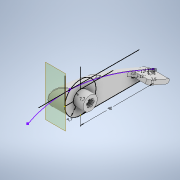
# Autodesk Inventor part: rachag2
Saved by Autodesk Inventor 2020 (Build 240168000, 168)
## iProperties
Created: 2023-10-21
Part Number: rachag2
Material: Типовые
Document SubType Name: Modeling
Designer: 522
Density: 1 g/cm^3
Appearance: По умолчанию
Author: 522
Autodesk Inventor part; units mm, degrees
ref_plane "YZ Plane" through (0, 0, 0) normal (1, 0, 0) x (0, 1, 0)
ref_plane "XZ Plane" through (0, 0, 0) normal (0, 1, 0) x (-1, 0, 0)
ref_plane "XY Plane" through (0, 0, 0) normal (0, 0, 1) x (1, 0, 0)
sketch "Эскиз1" plane through (0, 0, 0) normal (1, 0, 0) x (0, 1, 0)
  circle A0 centre (0, 0) radius 3.85
  circle A1 centre (0, 0) radius 8.55
  line L0 (-8.55, 0) -> (-8.55, -40)
  line L1 (6.55, 5.6577) -> (6.55, -32.1821)
  line L2 (3.85, 0) -> (3.85, -17.9751)
  line L3 (0, 0) -> (14.53, 0)
  line L4 (0, 0) -> (0, 8.55)
  line L5 (14.53, 8.55) -> (0, 8.55)
  arc A2 (-5.4255, -37.1668) -> (-6.7329, -39.9987) centre (-6.8, -38.25) ccw
  line L6 (6.55, 1.7425) -> (6.55, 23.1247)
  spline S0 degree 2 poles (-6.7329, -39.9987) (14.5192, 5.2155) (1.7917, 28.8286) knots 0 0 0 1 1 1
  line L7 (-6.8, -38.25) -> (-7.9249, -39.5906)
  line L8 (-6.8, -38.25) -> (-5.05, -38.25) construction
  line L9 (-1.9372, -28.9987) -> (-3.8265, -28.3121)
  line L10 (-1.9372, -28.9987) -> (-4.0049, -28.2473)
  line L11 (-6.7329, -39.9987) -> (-8.496, -38.6813)
  line L12 (-8.496, -38.6813) -> (-4.0049, -28.2473)
  point P0 (5.9063, 6.1821)
  point P1 (6.505, 5.5486)
  point P2 (-8.55, -38.25)
  point P3 (3.85, -11.5167)
  point P4 (3.85, -7.6341)
  point P5 (4.8879, -7.0151)
  dimension "d0" = 7.7
  dimension "d1" = 4.7
  dimension "d4" = 2.7
  dimension "d100" = 40
  dimension "d101" = 3.5
  dimension "d102" = 1.75
  dimension "d103" = 1.75
  dimension "d113" = 1.75
  dimension "d114" = 130
  dimension "d115" = 12
  dimension "d116" = 12
  dimension "d117" = 2.2
  constraints: 26 end point, 7 point on circle, 6 vertical, 2 centre point, 2 coincident, 2 horizontal, 2 point on line, 2 tangent, 1 equal length, 1 horizontal alignment, 1 perpendicular, 8 other
  measures "d4" distance between parallel lines of L2 L1
  measures "d100" distance of L0.start L0.end
  measures "d101" diameter of A2
  measures "d102" horizontal distance of L0.end L7.start
  measures "d103" horizontal distance of L0.end L7.start
  measures "d113" distance of L7.start L7.end
  measures "d114" angle of L7 L8
  measures "d115" distance of L7.end L9.end
  measures "d116" distance of L11.start L9.start
  measures "d117" distance of L9.start L10.end
extrude "Выдавливание1" add sketch "Эскиз1" against normal blind 10 contours L3 L4 A0 | L2 A1 L4 A0 | L3 S0 A1 L2 | A0 L4 L3 | A0 L4 A1 S0 L3 | L2 S0 L9 L10 L12 A2 L0 A1 | A1 S0 L2 | A2 L12 | S0 A2 L12 L10 L9 | A2 S0 L11 L12 | L11 L7 A2 | L7 L11 A2
sketch "Эскиз2" plane through (0, 0, 0) normal (1, 0, 0) x (0, 0, -1)
  line L0 (0, 0) -> (0, 14.4854)
  line L1 (0, 14.4854) -> (-8.5902, 14.4854)
  line L2 (-8.5902, 14.4854) -> (-8.55, -0.0237)
  arc A0 (-5.5486, 6.505) -> (0, -8.55) centre (0, 0) ccw projected
  point P0 (0, 8.55)
  point P1 (0, 8.55)
  point P2 (0, 8.55)
  point P3 (0, 8.55)
  constraints: 6 end point, 1 perpendicular, 1 point on circle, 1 tangent, 1 vertical
ref_plane "РабПлоскость1" through (0, 14.53, 8.55) normal (0, 0, -1) x (-1, 0, 0)
sketch "Эскиз5" plane through (0, 0, 0) normal (1, 0, 0) x (0, 0, -1)
  circle A0 centre (0, 0) radius 3.85
  line L0 (-11.3638, -1.8204) -> (-10.1238, -1.8204)
  line L1 (-10.1238, -1.8204) -> (-10.1238, -2.8204)
  line L2 (-10.1238, -2.8204) -> (-11.3638, -2.8204)
  line L3 (-11.3638, -2.8204) -> (-11.3638, -1.8204)
  line L4 (-11.3638, -1.8204) -> (-10.1238, -2.8204) construction
  line L5 (-10.1238, -1.8204) -> (-11.3638, -2.8204) construction
  line L6 (-10.6834, -1.8204) -> (-10.1238, -2.1204)
  line L7 (-10.6834, -2.8204) -> (-10.1238, -2.5204)
  circle A1 centre (0, 0) radius 2.1
  circle A2 centre (0, 0) radius 1.5
  line L8 (-2.3897, 1.3525) -> (-1.7469, 2.1185)
  line L9 (-1.7469, 2.1185) -> (-0.8277, 1.3472)
  line L10 (-0.8277, 1.3472) -> (-1.4705, 0.5812)
  line L11 (-1.4705, 0.5812) -> (-2.3897, 1.3525)
  line L12 (-2.3897, 1.3525) -> (-0.8277, 1.3472) construction
  line L13 (-1.7469, 2.1185) -> (-1.4705, 0.5812) construction
  line L14 (-1.241, 1.6941) -> (-1.0205, 1.1174)
  line L15 (-1.8838, 0.928) -> (-1.2776, 0.811)
  line L16 (-1.2385, -0.9829) -> (-2.3662, -1.3933)
  line L17 (-1.7456, -1.1674) -> (-1.3411, -0.701)
  line L18 (-2.3662, -1.3933) -> (-2.7082, -0.4536)
  line L19 (-2.7082, -0.4536) -> (-1.2385, -0.9829) construction
  line L20 (-2.0876, -0.2277) -> (-1.4779, -0.3251)
  line L21 (-1.5805, -0.0432) -> (-1.2385, -0.9829)
  line L22 (-2.3662, -1.3933) -> (-1.5805, -0.0432) construction
  line L23 (-2.7082, -0.4536) -> (-1.5805, -0.0432)
  line L24 (0.2319, -1.564) -> (0.0236, -2.7458)
  line L25 (0.1382, -2.0954) -> (-0.0635, -1.5119)
  line L26 (0.0236, -2.7458) -> (-0.9613, -2.5722)
  line L27 (-0.9613, -2.5722) -> (0.2319, -1.564) construction
  line L28 (-0.8466, -1.9218) -> (-0.4574, -1.4425)
  line L29 (-0.7529, -1.3904) -> (0.2319, -1.564)
  line L30 (0.0236, -2.7458) -> (-0.7529, -1.3904) construction
  line L31 (-0.9613, -2.5722) -> (-0.7529, -1.3904)
  line L32 (1.4705, -0.5812) -> (2.3897, -1.3525)
  line L33 (1.8838, -0.928) -> (1.2776, -0.811)
  line L34 (2.3897, -1.3525) -> (1.7469, -2.1185)
  line L35 (1.7469, -2.1185) -> (1.4705, -0.5812) construction
  line L36 (1.241, -1.6941) -> (1.0205, -1.1174)
  line L37 (0.8277, -1.3472) -> (1.4705, -0.5812)
  line L38 (2.3897, -1.3525) -> (0.8277, -1.3472) construction
  line L39 (1.7469, -2.1185) -> (0.8277, -1.3472)
  line L40 (1.2385, 0.9829) -> (2.3662, 1.3933)
  line L41 (1.7456, 1.1674) -> (1.3411, 0.701)
  line L42 (2.3662, 1.3933) -> (2.7082, 0.4536)
  line L43 (2.7082, 0.4536) -> (1.2385, 0.9829) construction
  line L44 (2.0876, 0.2277) -> (1.4779, 0.3251)
  line L45 (1.5805, 0.0432) -> (1.2385, 0.9829)
  line L46 (2.3662, 1.3933) -> (1.5805, 0.0432) construction
  line L47 (2.7082, 0.4536) -> (1.5805, 0.0432)
  line L48 (-0.2319, 1.564) -> (-0.0236, 2.7458)
  line L49 (-0.1382, 2.0954) -> (0.0635, 1.5119)
  line L50 (-0.0236, 2.7458) -> (0.9613, 2.5722)
  line L51 (0.9613, 2.5722) -> (-0.2319, 1.564) construction
  line L52 (0.8466, 1.9218) -> (0.4574, 1.4425)
  line L53 (0.7529, 1.3904) -> (-0.2319, 1.564)
  line L54 (-0.0236, 2.7458) -> (0.7529, 1.3904) construction
  line L55 (0.9613, 2.5722) -> (0.7529, 1.3904)
  point P0 (-10.7438, -2.3204)
  point P1 (-1.6087, 1.3499)
  point P2 (-1.9734, -0.7182)
  point P3 (-0.3647, -2.0681)
  point P4 (1.6087, -1.3499)
  point P5 (1.9734, 0.7182)
  point P6 (0.3647, 2.0681)
  point P7 (-1.241, 1.6941)
  point P8 (-0.1382, 2.0954)
  point P9 (0.8466, 1.9218)
  point P10 (1.7456, 1.1674)
  point P11 (2.0876, 0.2277)
  point P12 (1.8838, -0.928)
  point P13 (1.241, -1.6941)
  point P14 (0.1382, -2.0954)
  point P15 (-0.8466, -1.9218)
  point P16 (-1.7456, -1.1674)
  point P17 (-2.0876, -0.2277)
  point P18 (-1.8838, 0.928)
  point P19 (-1.7456, -1.1674)
  point P20 (-2.0876, -0.2277)
  dimension "d17" = 7.7
  dimension "d18" = 1
  dimension "d19" = 0.3
  dimension "d20" = 0.3
  dimension "d21" = 0.62
  dimension "d22" = 4.2
  dimension "d23" = 3
  dimension "d24" = 1
  dimension "d25" = 0.3
  dimension "d26" = 0.3
  dimension "d29" = 360
  constraints: 112 end point, 28 point on line, 14 midpoint, 4 parallel, 3 centre point, 3 coincident, 2 perpendicular, 1 horizontal, 103 other
  measures "d17" diameter of A0
  measures "d18" distance between parallel lines of L2 L0
  measures "d19" distance from line of L2 L7.end
  measures "d20" distance from line of L6.end L0
  measures "d21" distance from line of point (-10.744, -2.32) L1
  measures "d22" diameter of A1
  measures "d23" diameter of A2
  measures "d24" distance of L8.start L8.end
  measures "d25" distance of L9.end L14.end
  measures "d26" distance of L15.end L10.end
extrude "Выдавливание4" add sketch "Эскиз5" along normal blind 5.5 contours A0 | L44 L45 L41 A1 | A1 L40 L42 L47 | L32 L34 L39 A1 | A1 L36 L37 L33 | L52 L53 L49 A1 | A1 L48 L50 L55 | L24 L26 L31 A1 | A1 L28 L29 L25 | L14 L10 L15 A1 | A1 L11 L8 L9 | L16 L18 L23 A1 | A1 L20 L21 L17
extrude "Выдавливание5" cut sketch "Эскиз5" against normal blind 5 contours A1 L32 L37 A2 L45 L47 | L47 L45 L44 | L33 L37 L32 | L40 L45 A2 L53 L55 A1 | L41 L45 L40 | L39 L37 L36 | A1 L24 L29 A2 L37 L39 | L55 L53 L52 | A2 | L25 L29 L24 | L48 L53 A2 L10 L9 A1 | L49 L53 L48 | L31 L29 L28 | A1 L16 L21 A2 L29 L31 | L9 L10 L14 | A2 L21 L23 A1 L11 L10 | L16 L18 L23 A1 | L17 L21 L16 | L15 L10 L11 | L23 L21 L20
sketch "Эскиз16" plane through (0, 14.53, 8.55) normal (0, 0, -1) x (-1, 0, 0)
  point P0 (0, -14.53)
sketch "Эскиз18" plane through (0, -8.55, -38.25) normal (0, -1, 0) x (1, 0, 0)
  point P0 (0, 38.25)
sketch "Эскиз20" plane through (0, -8.55, -38.25) normal (0, -1, 0) x (1, 0, 0)
  line L0 (-10, 46.8) -> (-10, 38.25) projected
  line L1 (0, -1.7487) -> (0, 0) projected
  line L2 (-10, 46.8) -> (0, 46.8)
  line L3 (0, 46.8) -> (0, -1.7487)
  line L4 (0, -1.7487) -> (-10, -1.7487)
  line L5 (-10, -1.7487) -> (-10, 46.8)
  line L6 (0, -1.7487) -> (-10, -1.7487) projected
  line L7 (0, -1.7487) -> (-3.5, -1.7487)
  line L8 (0, 38.25) -> (0, 46.8) projected
  line L9 (-10, -1.7487) -> (0, 46.8)
  line L10 (-3.5, -1.7487) -> (-8.5061, 5.5042) construction
  line L11 (-8.5061, 5.5042) -> (-10, 46.8) construction
  spline S0 degree 2 poles (-3.5, -1.7487) (-8.5061, 5.5042) (-10, 46.8) knots 1 1 1 2 2 2
  point P0 (-10, 43.7986)
  point P1 (0, 43.7986)
  dimension "d109" = 3.5
  constraints: 12 end point, 2 parallel, 2 point on line, 1 horizontal, 1 perpendicular, 3 other
  measures "d109" distance of L1.start L7.end
extrude "Выдавливание12" [suppressed]
fillet "Сопряжение13" radius 9.75 3 edges at (-10, 4.4001, -9.2461) (-10, 5.9776, -0.5545) (-10, -0.4415, -25.1221)
extrude "Выдавливание13" add sketch "Эскиз1" along normal blind 9 contours S0 A2 L12 L10 L9 | A2 S0 L11 L12 | L11 L7 A2 | L7 L11 A2
fillet "Сопряжение14" radius 2.75 1 edges at (0, -2.9711, -28.623)
fillet "Сопряжение15" radius 1.5 1 edges at (9, -2.9711, -28.623)
fillet "Сопряжение16" radius 0.5 8 edges at (-10, -8.55, -9.4304) (-10, -7.0848, 4.7863) (-6.5694, 4.2298, 7.4304) (-0.125, 6.505, 5.5486) (-3.8063, -7.4221, -39.8857) (-0.125, -6.7329, -39.9987) (4.5, -6.7329, -39.9987) (-9.3751, -8.55, -28.496)
equation "\"d19\" = d20"
equation "\"d26\" = d25"
